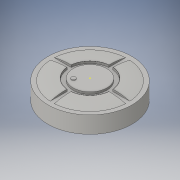
# Autodesk Inventor part: Simon
Saved by Autodesk Inventor 2016 (Build 200138000, 138)
## iProperties
Created: 2016-02-08
Part Number: Simon
Material: Generic
Document SubType Name: Modeling
Designer: yoruichin
Density: 1 g/cm^3
Appearance: Default
Author: yoruichin
Autodesk Inventor part; units mm, degrees
ref_plane "YZ Plane" through (0, 0, 0) normal (1, 0, 0) x (0, 1, 0)
ref_plane "XZ Plane" through (0, 0, 0) normal (0, 1, 0) x (-1, 0, 0)
ref_plane "XY Plane" through (0, 0, 0) normal (0, 0, 1) x (1, 0, 0)
sketch "Sketch1" plane through (0, 0, 0) normal (0, 1, 0) x (-1, 0, 0)
  circle A0 centre (0, 0) radius 100
  dimension "d0" = 200
  constraints: 1 centre point, 1 coincident
  measures "d0" diameter of A0
extrude "Extrusion1" add sketch "Sketch1" along normal blind 40
sketch "Sketch2" plane through (0, 40, 0) normal (0, 1, 0) x (1, 0, 0)
  circle A0 centre (0, 0) radius 90
  dimension "d3" = 180
  constraints: 1 centre point, 1 coincident
  measures "d3" diameter of A0
extrude "Extrusion2" add sketch "Sketch2" along normal blind 5
sketch "Sketch3" plane through (0, 45, 0) normal (0, 1, 0) x (1, 0, 0)
  point P0 (0, 0)
sketch "Sketch4" plane through (0, 45, 0) normal (0, 1, 0) x (1, 0, 0)
  point P0 (0, 0)
sketch "Sketch5" plane through (0, 45, 0) normal (0, 1, 0) x (1, 0, 0)
  line L0 (-5, -90) -> (5, -90)
  line L1 (5, -90) -> (5, 90)
  line L2 (5, 90) -> (-5, 90)
  line L3 (-5, 90) -> (-5, -90)
  line L4 (-5, -90) -> (5, 90) construction
  line L5 (5, -90) -> (-5, 90) construction
  point P0 (0, 0)
  dimension "d6" = 10
  dimension "d7" = 180
  constraints: 12 end point, 2 midpoint, 2 parallel, 1 horizontal, 1 perpendicular
  measures "d6" distance of L2.end L1.end
  measures "d7" distance of L1.end L0.end
extrude "Extrusion3" cut sketch "Sketch5" against normal blind 5
sketch "Sketch6" plane through (0, 45, 0) normal (0, 1, 0) x (1, 0, 0)
  line L0 (-90, 5) -> (90, 5)
  line L1 (90, 5) -> (90, -5)
  line L2 (90, -5) -> (-90, -5)
  line L3 (-90, -5) -> (-90, 5)
  line L4 (-90, 5) -> (90, -5) construction
  line L5 (90, 5) -> (-90, -5) construction
  point P0 (0, 0)
  dimension "d10" = 180
  dimension "d11" = 10
  constraints: 12 end point, 2 midpoint, 2 parallel, 1 horizontal, 1 perpendicular
  measures "d10" distance of L1.end L2.end
  measures "d11" distance of L0.end L1.end
extrude "Extrusion4" cut sketch "Sketch6" against normal blind 5
sketch "Sketch7" plane through (0, 40, 0) normal (0, 1, 0) x (1, 0, 0)
  point P0 (0, 0)
sketch "Sketch8" plane through (0, 40, 0) normal (0, 1, 0) x (1, 0, 0)
  circle A0 centre (0, 0) radius 50
  dimension "d14" = 100
  constraints: 1 centre point, 1 coincident
  measures "d14" diameter of A0
extrude "Extrusion6" cut sketch "Sketch8" along normal blind 10
sketch "Sketch10" plane through (0, 40, 0) normal (0, 1, 0) x (1, 0, 0)
  circle A0 centre (0, 0) radius 40
  dimension "d20" = 80
  constraints: 1 centre point, 1 coincident
  measures "d20" diameter of A0
extrude "Extrusion7" add sketch "Sketch10" along normal blind 5
sketch "Sketch11" plane through (0, 0, 0) normal (0, -1, 0) x (1, 0, 0)
  circle A0 centre (85, 0) radius 7.5
  point P0 (0, 0)
  dimension "d23" = 15
  constraints: 1 centre point
  measures "d23" diameter of A0
extrude "Extrusion8" add sketch "Sketch11" along normal blind 5
pattern_circular "Circular Pattern1" count 6 over 360 about axis through (0, 0, 0) along (0, 1, 0) of "Extrusion8", "Extrusion1", "Extrusion7"
fillet "Fillet1" radius 159.1625 4 edges at (63.6396, 45, 63.6396) (-63.6396, 45, 63.6396) (-63.6396, 45, -63.6396) (63.6396, 45, -63.6396)
sketch "Sketch12" plane through (0, 45, 0) normal (0, 1, 0) x (1, 0, 0)
  point P0 (0, 0)
sketch "Sketch13" plane through (0, 45, 0) normal (0, 1, 0) x (1, 0, 0)
  circle A0 centre (-18.2246, -20.9627) radius 5
  point P0 (0, 0)
  dimension "d30" = 10
  constraints: 1 centre point
  measures "d30" diameter of A0
extrude "Extrusion9" add sketch "Sketch13" along normal mid plane 3
body "Solid1"
